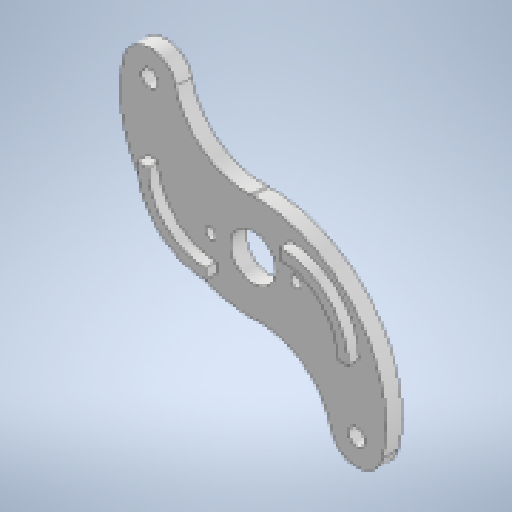
# Autodesk Inventor part: rotor
Saved by Autodesk Inventor 2024.3 (Build 283343010, 343A)
## iProperties
Created: 2025-06-26
Part Number: rotor
Material: 一般
Document SubType Name: Modeling
Designer: kshau
Density: 1 g/cm^3
Appearance: 既定
Author: kshau
Autodesk Inventor part; units mm, degrees
ref_plane "YZ Plane" through (0, 0, 0) normal (1, 0, 0) x (0, 1, 0)
ref_plane "XZ Plane" through (0, 0, 0) normal (0, 1, 0) x (-1, 0, 0)
ref_plane "XY Plane" through (0, 0, 0) normal (0, 0, 1) x (1, 0, 0)
sketch "スケッチ1" plane through (0, 0, 0) normal (0, 0, 1) x (1, 0, 0)
  circle A0 centre (0, 0) radius 27.5
  line L0 (0, 27.5) -> (0, 0)
  line L1 (8, 0) -> (19.4453, -19.4456)
  line L2 (0, 0) -> (27.5, 0)
  circle A1 centre (19.4453, -19.4456) radius 5
  circle A2 centre (0, 0) radius 10
  arc A3 (24.3161, -20.5748) -> (0, 10) centre (0.0187, -14.9418) ccw
  line L3 (24.3161, -20.5748) -> (14.5745, -20.5748)
  arc A4 (14.5745, -20.5748) -> (0.5179, -9.9866) centre (1.2275, -23.6691) ccw
  arc A5 (-24.3161, 20.5748) -> (0, -10) centre (-0.0187, 14.9418) ccw
  arc A6 (-14.5745, 20.5748) -> (-0.5179, 9.9866) centre (-1.2275, 23.6691) ccw
  circle A7 centre (-19.4453, 19.4456) radius 5
  point P0 (-0.5179, 9.9866)
  point P1 (0, -10)
  point P2 (0, 10)
  dimension "d4" = 20
  dimension "d0" = 55
  dimension "d1" = 8
  dimension "d2" = 22.5638
  dimension "d3" = 10
  dimension "d5" = 9.7416
  dimension "d9" = 360
  constraints: 15 point on circle, 8 end point, 7 centre point, 3 coincident, 2 tangent, 1 horizontal, 1 parallel, 1 point on line, 1 vertical, 26 other
  measures "d0" diameter of A0
  measures "d1" distance from line of L0 L1.start
  measures "d2" distance of L1.start L1.end
  measures "d3" diameter of A1
  measures "d5" distance of L3.start L3.end
extrude "押し出し1" add sketch "スケッチ1" along normal blind 3 contours A3 A1 A0 | A0 A1 L1 A2 L2 A3 | L2 A2 A3 | A7 A0 | A0 A7 | A2 L2 L0 | L0 L2 L1 A2 | A1 L3 A0 | A0 L1 A1 | A1 A0 L3 | A2 L1 L2 | A7 A6 A2 A5 A0 | A0 A5 A7 | A0 L3 A1 L1 | A1 A4 A2 L1 | A1 L3 A0
sketch "スケッチ2" plane through (0, 0, 3) normal (0, 0, 1) x (1, 0, 0)
  circle A0 centre (0, 0) radius 4.25
  dimension "d13" = 8.5
  constraints: 1 centre point, 1 coincident
  measures "d13" diameter of A0
extrude "押し出し2" cut sketch "スケッチ2" against normal blind 3
sketch "スケッチ3" plane through (0, 0, 3) normal (0, 0, 1) x (1, 0, 0)
  arc A0 (-14.5745, 20.5748) -> (-24.3161, 20.5748) centre (-19.4453, 19.4456) ccw projected
  arc A1 (14.5745, -20.5748) -> (24.3161, -20.5748) centre (19.4453, -19.4456) ccw projected
  circle A2 centre (0, 0) radius 4.25 projected
  point P0 (8, 0)
  point P1 (-8, 0)
  dimension "d16" = 8
  dimension "d17" = 8
  constraints: 2 coincident
  measures "d16" distance of A2.centre point (8, 0)
  measures "d17" distance of A2.centre point (-8, 0)
hole "穴1" at (-19.4453, 19.4456, 3) at (19.4453, -19.4456, 3) at (8, 0, 3) at (-8, 0, 3) direction (0, 0, -1) diameter 2 end through all
sketch "スケッチ4" plane through (0, 0, 3) normal (0, 0, 1) x (1, 0, 0)
  circle A0 centre (0, 0) radius 9.289
  circle A1 centre (8, 0) radius 1 projected
  circle A2 centre (8, 0) radius 6.227
  circle A3 centre (0, 0) radius 8.107
  circle A4 centre (8, 0) radius 4.2674
  line L0 (6.9694, 6.1411) -> (6.9695, 4.1411)
  circle A5 centre (6.9703, -6.6969) radius 12.838
  circle A6 centre (0, 0) radius 20.909
  circle A7 centre (8, 0) radius 13.574
  line L1 (19.8083, -6.6946) -> (17.8083, -6.6948)
  arc A8 (17.8083, -6.6948) -> (6.9695, 4.1411) centre (6.9703, -6.6969) ccw
  circle A9 centre (-6.9703, 6.6969) radius 12.838
  line L2 (-19.8083, 6.6946) -> (-17.8083, 6.6948)
  arc A10 (-17.8083, 6.6948) -> (-6.9695, -4.1411) centre (-6.9703, 6.6969) ccw
  line L3 (-6.9694, -6.1411) -> (-6.9695, -4.1411)
  point P0 (6.9695, 4.1411)
  point P1 (-6.9695, -4.1411)
  dimension "d25" = 18.578
  dimension "d26" = 12.454
  dimension "d30" = 41.818
  dimension "d31" = 27.148
  dimension "d27" = 16.214
  dimension "d29" = 25.676
  dimension "d32" = 2
  dimension "d33" = 2
  dimension "d36" = 360
  constraints: 10 point on circle, 8 coincident, 8 end point, 5 centre point, 1 perpendicular, 38 other
  measures "d27" diameter of A3
  measures "d29" diameter of A5
  measures "d32" distance of L0.start L0.end
  measures "d33" distance of L1.start L1.end
extrude "押し出し3" add sketch "スケッチ4" along normal blind 2 contours A8 A4 A0 | A0 A4 A8 | A4 L0 A0 | A0 A5 A2 A8 A4 | A2 A5 L1 A8 | A9 L2 A10 A0 | A0 A10 L3 picked at (7.7179, 4.1654) picked at (9.1795, 4.0223)
sketch "スケッチ5" plane through (0, 0, 0) normal (0, 0, -1) x (-1, 0, 0)
  circle A0 centre (19.4453, 19.4456) radius 1 projected
  circle A1 centre (-19.4453, -19.4456) radius 1 projected
  point P0 (0, 0)
  constraints: 2 coincident
hole "穴2" at (-19.4453, 19.4456, 0) at (19.4453, -19.4456, 0) direction (0, 0, 1) diameter 3.1 end through all
